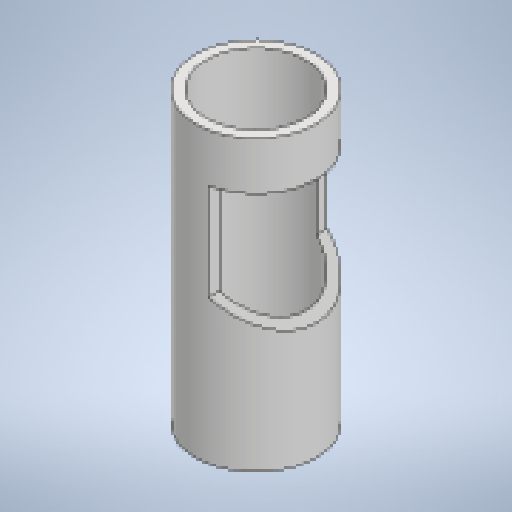
# Autodesk Inventor part: NVPH-404 second tube
Saved by Autodesk Inventor 2025 (Build 290162010, 162A)
## iProperties
Created: 2024-12-03
Part Number: NVPH-404 second tube
Material: Generic
Document SubType Name: Modeling
Designer: user
Density: 1 g/cm^3
Appearance: Default
Author: user
Autodesk Inventor part; units mm, degrees
ref_plane "YZ Plane" through (0, 0, 0) normal (1, 0, 0) x (0, 1, 0)
ref_plane "XZ Plane" through (0, 0, 0) normal (0, 1, 0) x (-1, 0, 0)
ref_plane "XY Plane" through (0, 0, 0) normal (0, 0, 1) x (1, 0, 0)
sketch "Sketch1" plane through (0, 0, 0) normal (0, 0, 1) x (1, 0, 0)
  circle A0 centre (0, 0) radius 52
  circle A1 centre (0, 0) radius 62.5
  dimension "d0" = 125
  dimension "d1" = 104
  constraints: 2 centre point, 2 coincident
  measures "d0" diameter of A1
  measures "d1" diameter of A0
extrude "Extrusion1" add sketch "Sketch1" along normal blind 400
sketch "Sketch2" plane through (0, 0, 0) normal (0, 1, 0) x (-1, 0, 0)
  line L0 (62.5, 400) -> (-62.5, 400) projected
  line L1 (62.5, 0) -> (-62.5, 0) projected
  line L2 (-62.5, 280) -> (-12.5, 280)
  line L3 (-12.5, 280) -> (-12.5, 210)
  line L4 (-12.5, 210) -> (-62.5, 181.1325)
  line L5 (-62.5, 0) -> (-62.5, 400) projected
  point P0 (0, 0)
  dimension "d4" = 60
  dimension "d5" = 50
  dimension "d6" = 120
  dimension "d7" = 70
  constraints: 6 end point, 2 point on line, 1 horizontal, 1 perpendicular
  measures "d4" angle of L5 L4
  measures "d5" distance of L2.start L2.end
  measures "d6" distance between parallel lines of L2 L0
  measures "d7" distance of L2.end L3.end
extrude "Extrusion2" cut sketch "Sketch2" along normal through all both and the other way through all
body "Solid1"
